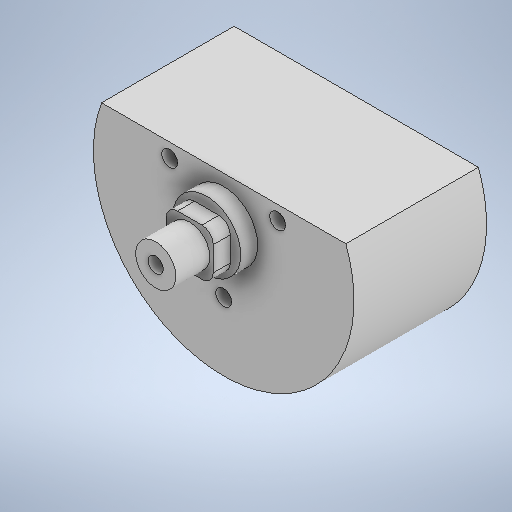
# Autodesk Inventor part: WheelSupportTemp
Saved by Autodesk Inventor 2025.1 (Build 291241000, 241)
## iProperties
Created: 2025-04-04
Part Number: WheelSupportTemp
Material: Generic
Document SubType Name: Modeling
Designer: victo
Density: 1 g/cm^3
Appearance: Default
Author: victo
Autodesk Inventor part; units mm, degrees
ref_plane "YZ Plane" through (0, 0, 0) normal (1, 0, 0) x (0, 1, 0)
ref_plane "XZ Plane" through (0, 0, 0) normal (0, 1, 0) x (-1, 0, 0)
ref_plane "XY Plane" through (0, 0, 0) normal (0, 0, 1) x (1, 0, 0)
sketch "Sketch1" plane through (0, 0, 0) normal (0, 0, 1) x (1, 0, 0)
  circle A0 centre (0, 0) radius 23
  line L0 (-21.5639, 8) -> (21.5639, 8)
  dimension "d0" = 46
  dimension "d1" = 8
  constraints: 2 end point, 2 point on circle, 1 centre point, 1 coincident, 1 horizontal
  measures "d0" diameter of A0
  measures "d1" distance from line of L0 point (0, 0)
extrude "Extrusion1" add sketch "Sketch1" along normal blind 23.4 contours A0 L0 picked at (2.2543, -4.6669)
sketch "Sketch2" plane through (0, 0, 23.4) normal (0, 0, 1) x (1, 0, 0)
  circle A0 centre (0, 0) radius 6
  dimension "d4" = 12
  constraints: 1 centre point, 1 coincident
  measures "d4" diameter of A0
extrude "Extrusion2" add sketch "Sketch2" along normal blind 3
sketch "Sketch3" plane through (0, 0, 26.4) normal (0, 0, 1) x (1, 0, 0)
  line L0 (-4.15, 4.15) -> (4.15, 4.15)
  line L1 (4.15, 4.15) -> (4.15, -4.15)
  line L2 (4.15, -4.15) -> (-4.15, -4.15)
  line L3 (-4.15, -4.15) -> (-4.15, 4.15)
  line L4 (-4.15, 4.15) -> (4.15, -4.15) construction
  line L5 (4.15, 4.15) -> (-4.15, -4.15) construction
  point P0 (0, 0)
  dimension "d7" = 8.3
  dimension "d8" = 8.3
  constraints: 12 end point, 2 midpoint, 2 parallel, 1 horizontal, 1 perpendicular
  measures "d7" distance between parallel lines of L3 L1
  measures "d8" distance between parallel lines of L0 L2
extrude "Extrusion3" add sketch "Sketch3" along normal blind 3
fillet "Fillet1" radius 2 4 edges at (4.15, 4.15, 27.9) (4.15, -4.15, 27.9) (-4.15, -4.15, 27.9) (-4.15, 4.15, 27.9)
sketch "Sketch4" plane through (0, 0, 29.4) normal (0, 0, 1) x (1, 0, 0)
  circle A0 centre (0, 0) radius 3.55
  dimension "d12" = 7.1
  constraints: 1 centre point, 1 coincident
  measures "d12" diameter of A0
extrude "Extrusion4" add sketch "Sketch4" along normal blind 6
sketch "Sketch5" plane through (0, 0, 35.4) normal (0, 0, 1) x (1, 0, 0)
  circle A0 centre (0, 0) radius 1.35
  dimension "d15" = 2.7
  constraints: 1 centre point, 1 coincident
  measures "d15" diameter of A0
extrude "Extrusion5" cut sketch "Sketch5" against normal blind 10
sketch "Sketch6" plane through (0, 0, 23.4) normal (0, 0, 1) x (1, 0, 0)
  circle A0 centre (0, -11) radius 1.4
  circle A1 centre (0, 0) radius 1.35 projected
  circle A2 centre (9.5263, 5.5) radius 1.4
  circle A3 centre (-9.5263, 5.5) radius 1.4
  dimension "d18" = 2.8
  dimension "d19" = 11
  dimension "d22" = 360
  constraints: 3 centre point, 7 other
  measures "d18" diameter of A0
  measures "d19" distance of point (0, 0) A0.centre
extrude "Extrusion6" cut sketch "Sketch6" against normal blind 10 contours A0 | A2 | A3
equation "\"d8\" = d7"
body "Solid1"
